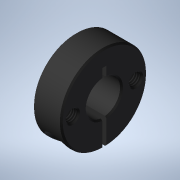
# Autodesk Inventor part: SCSW12-10b
Saved by Autodesk Inventor 2021 (Build 250183000, 183)
## iProperties
Created: 2025-01-13
Part Number: SCSW12-10b
Material: Generic
Catalog Web Link: www.cadenas.de
Description: SCSW, PSCSW, SSCSW, SCSWA, SCSWAW-b-Set Collars - Slit 2 Hole/2 Tap - Standard Type - 2 Tap Type
Vendor: MISUMI
Document SubType Name: Modeling
Designer: psAdmin
Manufacturer: MISUMI
Mass: 5.03092 g
Surface Area: 30.3067 cm^2
Volume: 5.03092 cm^3
Density: 1 g/cm^3
Appearance: PSOLRGB-175-175-175
Category: PARTsolutions
Company: MISUMI
Title: SCSW12-10b
Author: Cadenas PARTsolutions
Comments: Set Collars - Slit 2 Hole/2 Tap - Standard Type - 2 Tap Type
PSOL_IDENT_0: {$CADENAS_DATA/23d-libs/misumi/metric/03_set_collars/scsw_b.prj},200 {VTYP=3D},{NB=SCSW12-10b},{LINA=
PSOL_IDENT_1: SCSW12-10b},{NN=SCSW, PSCSW, SSCSW, SCSWA, SCSWAW-b},{DATE=29.11.2024 04:05:21},{GEOMDATE=15.09.2021
PSOL_IDENT_2: 06:01:21},{VERSION=},{LINEID=70},{WBVAR=MAT,ST,BS},{WBNUMERIC=BS}  {NB=SCSW12-10b},{LINA=SCSW12-10b
PSOL_IDENT_3: },{KT=DUMMY},{PN=SCSW12-10},{TYPE=SCSW},{MAT=1045},{MATA='1045','S45C Equivalent','304','SUS304 Equi
PSOL_IDENT_4: valent','2017','2017 Aluminum Alloy'},{ST=Black Oxide},{AC=Hexagon Socket Head Set Screw 1 Pc.},{D=1
PSOL_IDENT_5: 2},{BS=10},{B1=8,10,12,15},{D1=30},{M=M4},{THMD=4},{THDMIN=3.242},{ST0='Black Oxide','Black Oxide','
PSOL_IDENT_6: Electroless Nickel Plating','Electroless Nickel Plating'},{DD=4.5},{R=3.75},{W=1.5},{X=10.0},{Y=5.0}
PSOL_IDENT_7: ,{Z=9~10},{S=5.5},{P=22},{C=0.5},{L=12},{M1=M5},{ZZ=9.5},{THMD1=5},{THDMIN1=4.134}
NB: SCSW12-10b
NN: SCSW, PSCSW, SSCSW, SCSWA, SCSWAW-b
NT: Set Collars - Slit 2 Hole/2 Tap - Standard Type - 2 Tap Type
NBSYN: $PN.b
LINA: SCSW12-10b
CATALOG: Misumi
PN: SCSW12-10
MAT: S45C Equivalent
ST: Black Oxide
AC: Hexagon Socket Head Set Screw 1 Pc.
D: 12
BS: 10
D1: 30
M: M4
DD: 4.5
R: 3.75
W: 1.5
X: 10
Y: 5
Z: 9~10
S: 5.5
P: 22
M1: M5
SUPPLIER: MISUMI
ARTICLENO: SCSW12-10b
BOMINFO: SCSW12-10b
CREATOR: CADENAS GmbH
Autodesk Inventor part; units mm, degrees
sketch "Sketch_1" plane through (0, 0, 0) normal (0, 0, 1) x (1, 0, 0)
  line L0 (5, 0) -> (-5, 0)
  line L1 (-5, 14.5) -> (-5, 6.5)
  line L2 (-5, 6.5) -> (-4.5, 6)
  line L3 (-4.5, 6) -> (4.5, 6)
  line L4 (4.5, 6) -> (5, 6.5)
  line L5 (5, 6.5) -> (5, 14.5)
  line L6 (5, 14.5) -> (4.5, 15)
  line L7 (4.5, 15) -> (-4.5, 15)
  line L8 (-4.5, 15) -> (-5, 14.5)
  constraints: 18 end point
revolve "Revolution1" add sketch "Sketch_1" angle 360 about axis through (5, 0, 0) along (1, 0, 0)
sketch "Sketch_2" plane through (0, 0, 0) normal (1, 0, 0) x (0, 1, 0)
  line L0 (-15, 0.75) -> (-15, -0.75)
  line L1 (-15, -0.75) -> (9.5, -0.75)
  line L2 (9.5, -0.75) -> (9.5, 0.75)
  line L3 (9.5, 0.75) -> (-15, 0.75)
  constraints: 8 end point
extrude "Extrusion1" cut sketch "Sketch_2" along normal mid plane 10
sketch "Sketch_3" plane through (0, 0, 0) normal (1, 0, 0) x (0, 1, 0)
  line L0 (-10, 15) -> (-10, 0)
  line L1 (-10, 0) -> (-12.25, 0)
  line L2 (-12.25, 0) -> (-12.25, 5)
  line L3 (-12.25, 5) -> (-13.75, 5)
  line L4 (-13.75, 5) -> (-13.75, 15)
  line L5 (-13.75, 15) -> (-10, 15)
  line L6 (-10, 15) -> (-10, 0)
  constraints: 14 end point
revolve "Revolution2" cut sketch "Sketch_3" angle 360 about axis through (0, -10, 15) along (0, 0, 1)
sketch "Sketch_4" plane through (0, 0, 0) normal (1, 0, 0) x (0, 1, 0)
  line L0 (-10, -15.75) -> (-10, -0.75)
  line L1 (-10, -0.75) -> (-8, -0.75)
  line L2 (-8, -0.75) -> (-8.379, -1.129)
  line L3 (-8.379, -1.129) -> (-8.379, -15.75)
  line L4 (-8.379, -15.75) -> (-10, -15.75)
  line L5 (-10, -15.75) -> (-10, -0.75)
  constraints: 12 end point
revolve "Revolution3" cut sketch "Sketch_4" angle 360 about axis through (0, -10, -15.75) along (0, 0, -1)
thread "Thread1" size "M4x0.7" class "6H" standard "ISO Metric profile" length 11.5596
sketch "Sketch_7" plane through (0, 0, -11) normal (0, 0, 1) x (1, 0, 0)
  line L0 (5, 0) -> (-5, 0)
  line L1 (-5, 0) -> (-5, 2.5)
  line L2 (-5, 2.5) -> (-4.567, 2.067)
  line L3 (-4.567, 2.067) -> (4.567, 2.067)
  line L4 (4.567, 2.067) -> (5, 2.5)
  line L5 (5, 2.5) -> (5, 0)
  line L6 (5, 0) -> (-5, 0)
  constraints: 14 end point
revolve "Revolution4" cut sketch "Sketch_7" angle 360 about axis through (5, 0, -11) along (1, 0, 0)
thread "Thread2" size "M5x0.8" class "6H" standard "ISO Metric profile" full length
sketch "Sketch_8" plane through (0, 0, 11) normal (0, 0, 1) x (1, 0, 0)
  line L0 (5, 0) -> (-5, 0)
  line L1 (-5, 0) -> (-5, 2.5)
  line L2 (-5, 2.5) -> (-4.567, 2.067)
  line L3 (-4.567, 2.067) -> (4.567, 2.067)
  line L4 (4.567, 2.067) -> (5, 2.5)
  line L5 (5, 2.5) -> (5, 0)
  line L6 (5, 0) -> (-5, 0)
  constraints: 14 end point
revolve "Revolution5" cut sketch "Sketch_8" angle 360 about axis through (5, 0, 11) along (1, 0, 0)
thread "Thread3" size "M5x0.8" class "6H" standard "ISO Metric profile" full length
ref_plane "body_screw_XY" through (0, -10, 5) normal (0, 0, 1) x (1, 0, 0)
ref_plane "body_screw_YZ" through (0, -10, 5) normal (1, 0, 0) x (0, 1, 0)
ref_plane "body_screw_ZX" through (0, -10, 5) normal (0, 1, 0) x (0, 0, 1)
body "Solid1"
